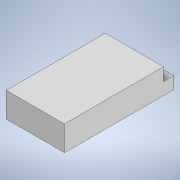
# Autodesk Inventor part: PowerSupply
Saved by Autodesk Inventor 2020 (Build 240168000, 168)
## iProperties
Created: 2020-04-19
Part Number: PowerSupply
Material: Типовые
Document SubType Name: Modeling
Designer: Михаил
Density: 1 g/cm^3
Appearance: По умолчанию
Author: Михаил
Autodesk Inventor part; units mm, degrees
ref_plane "YZ Plane" through (0, 0, 0) normal (1, 0, 0) x (0, 1, 0)
ref_plane "XZ Plane" through (0, 0, 0) normal (0, 1, 0) x (-1, 0, 0)
ref_plane "XY Plane" through (0, 0, 0) normal (0, 0, 1) x (1, 0, 0)
sketch "Эскиз1" plane through (0, 0, 0) normal (0, 1, 0) x (-1, 0, 0)
  line L0 (0, 0) -> (114, 0)
  line L1 (114, 0) -> (114, -214)
  line L2 (114, -214) -> (0, -214)
  line L3 (0, -214) -> (0, 0)
  dimension "d0" = 114
  dimension "d1" = 214
  constraints: 8 end point, 2 parallel, 1 horizontal, 1 perpendicular
  measures "d0" distance of L1.end L2.end
  measures "d1" distance of L0.end L1.end
extrude "Выдавливание1" add sketch "Эскиз1" along normal blind 49
sketch "Эскиз2" plane through (0, 49, 0) normal (0, 1, 0) x (1, 0, 0)
  line L0 (0, 0) -> (0, 214) projected
  line L1 (-114, 214) -> (-114, 0) projected
  line L2 (0, 214) -> (-114, 214)
  line L3 (-114, 214) -> (-114, 194)
  line L4 (-114, 194) -> (0, 194)
  line L5 (0, 194) -> (0, 214)
  dimension "d4" = 20
  constraints: 8 end point, 2 parallel, 1 horizontal, 1 perpendicular, 1 point on line
  measures "d4" distance of L3.end L2.end
extrude "Выдавливание2" cut sketch "Эскиз2" against normal blind 25
